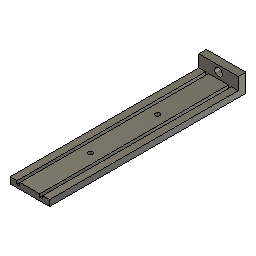
E Closer (Autodesk Fusion 360 design; units mm, degrees)
Autodesk Fusion 360 part; units mm, degrees
sketch "Eskiz1" plane through (0, 0, 0) normal (0, 1, 0) x (1, 0, 0)
  line L0 (0, 0) -> (26, 0)
  line L1 (26, 0) -> (26, -124)
  line L2 (26, -124) -> (0, -124)
  line L3 (0, -124) -> (0, 0)
  line L4 (4.5, 0) -> (6.5, 0)
  line L5 (6.5, 0) -> (6.5, -124)
  line L6 (6.5, -124) -> (4.5, -124)
  line L7 (4.5, -124) -> (4.5, 0)
  line L8 (19.5, 0) -> (21.5, 0)
  line L9 (21.5, 0) -> (21.5, -124)
  line L10 (21.5, -124) -> (19.5, -124)
  line L11 (19.5, -124) -> (19.5, 0)
  line L12 (0, 0) -> (26, 0)
  line L13 (26, 0) -> (26, 5)
  line L14 (26, 5) -> (0, 5)
  line L15 (0, 5) -> (0, 0)
  line L16 (0, -124) -> (26, -124)
  line L17 (26, -124) -> (26, -129)
  line L18 (26, -129) -> (0, -129)
  line L19 (0, -129) -> (0, -124)
  dimension "d1" = 26
  dimension "d2" = 124
  dimension "d3" = 2
  dimension "d4" = 4.5
  dimension "d5" = 2
  dimension "d6" = 13
  dimension "d11" = 5
  dimension "d18" = 5
  constraint horizontal L0
  constraint vertical L1
  constraint horizontal L2
  constraint vertical L3
  constraint coincident L0.start L3.end
  constraint horizontal L4
  constraint vertical L5
  constraint horizontal L6
  constraint vertical L7
  constraint coincident L0 L4.start
  constraint horizontal L8
  constraint vertical L9
  constraint horizontal L10
  constraint vertical L11
  constraint coincident L0 L8.start
  constraint horizontal L12
  constraint vertical L13
  constraint horizontal L14
  constraint vertical L15
  constraint horizontal L16
  constraint vertical L17
  constraint horizontal L18
  constraint vertical L19
  measures "d1" distance of L0.start L0.end
  measures "d2" distance of L0.start L2.end
  measures "d3" distance of L4.start L4.end
  measures "d4" distance of L0.start L4.start
  measures "d5" distance of L8.start L8.end
  measures "d6" distance of L4.end L8.start
  measures "d11" distance of L0.start L14.end
  measures "d18" distance of L2.end L18.end
extrude "Ekstrüde Et1" add sketch "Eskiz1" along normal blind 2 contours L0 L2 L4 L5 L6 L7 L12 L16 | L0 L2 L8 L9 L10 L11 L12 L16 makes body 1 at (6.5, 0.6667, 41.3333) makes body 2 at (21.5, 0.6667, 41.3333)
extrude "Ekstrüde Et2" add sketch "Eskiz1" along normal blind 4 contours L0 L2 L3 L7 L12 L16 | L0 L2 L5 L11 L12 L16 | L0 L1 L2 L9 L12 L16 bodies 1 2
extrude "Ekstrüde Et3" add sketch "Eskiz1" along normal blind 12 contours L0 L4 L8 L12 L13 L14 L15 bodies 1
sketch "Eskiz2" plane through (0, 0, -5) normal (0, 0, -1) x (-1, 0, 0)
  line L0 (-26, 0) -> (0, 0)
  line L1 (0, 0) -> (0, 12)
  line L2 (0, 12) -> (-26, 12)
  line L3 (-26, 12) -> (-26, 0)
  circle A0 centre (-13, 8) radius 2.5
  dimension "d14" = 5
  dimension "d15" = 4
  measures "d14" diameter of A0
  measures "d15" distance of L2 A0.centre
extrude "Ekstrüde Et4" cut sketch "Eskiz2" against normal blind 6 contours A0 bodies 1
sketch "Eskiz3" plane through (0, 4, 0) normal (0, 1, 0) x (-1, 0, 0)
  line L0 (-6.5, 0) -> (-6.5, 124)
  line L1 (-6.5, 124) -> (-19.5, 124)
  line L2 (-19.5, 124) -> (-19.5, 0)
  line L3 (-19.5, 0) -> (-6.5, 0)
  circle A0 centre (-13, 84) radius 1.5
  circle A1 centre (-13, 40) radius 1.5
  dimension "d19" = 3
  dimension "d20" = 3
  dimension "d21" = 40
  dimension "d22" = 40
  measures "d19" diameter of A0
  measures "d20" diameter of A1
  measures "d21" distance of L3 A1.centre
  measures "d22" distance of L1 A0.centre
extrude "Ekstrüde Et5" cut sketch "Eskiz3" against normal blind 15 contours A0 | A1 bodies 1
